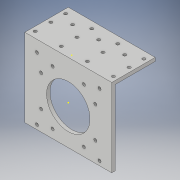
# Autodesk Inventor part: ousterholderm600V2
Saved by Autodesk Inventor 2019 (Build 230136000, 136)
## iProperties
Created: 2019-07-12
Part Number: ousterholderm600V2
Material: Generic
Document SubType Name: Modeling
Designer: Dell
Density: 1 g/cm^3
Appearance: Default
Author: Dell
Autodesk Inventor part; units mm, degrees
ref_plane "YZ Plane" through (0, 0, 0) normal (1, 0, 0) x (0, 1, 0)
ref_plane "XZ Plane" through (0, 0, 0) normal (0, 1, 0) x (-1, 0, 0)
ref_plane "XY Plane" through (0, 0, 0) normal (0, 0, 1) x (1, 0, 0)
sketch "Sketch3" plane through (0, 0, 0) normal (0, 0, 1) x (1, 0, 0)
  line L0 (-50, 45) -> (50, 45)
  line L1 (50, 45) -> (50, -45)
  line L2 (50, -45) -> (-50, -45)
  line L3 (-50, -45) -> (-50, 45)
  line L4 (-50, 45) -> (50, -45) construction
  line L5 (50, 45) -> (-50, -45) construction
  point P0 (0, 0)
  dimension "d4" = 100
  dimension "d5" = 90
  constraints: 12 end point, 2 midpoint, 2 parallel, 1 horizontal, 1 perpendicular
  measures "d4" distance of L1.end L2.end
  measures "d5" distance of L0.end L1.end
extrude "Extrusion2" add sketch "Sketch3" along normal blind 4
sketch "Sketch4" plane through (0, 0, 4) normal (0, 0, 1) x (1, 0, 0)
  point P0 (0, 0)
sketch "Sketch5" plane through (0, 0, 4) normal (0, 0, 1) x (1, 0, 0)
  line L0 (50, 45) -> (-50, 45) projected
  line L1 (50, 45) -> (-50, 45)
  line L2 (-50, 45) -> (-50, 41)
  line L3 (-50, 41) -> (50, 41)
  line L4 (50, 41) -> (50, 45)
  point P0 (0, 0)
  dimension "d8" = 4
  dimension "d9" = 100
  constraints: 8 end point, 2 parallel, 1 horizontal, 1 perpendicular
  measures "d8" distance of L1.end L2.end
  measures "d9" distance of L2.end L3.end
extrude "Extrusion3" add sketch "Sketch5" against normal blind 50
sketch "Sketch6" plane through (0, 0, 4) normal (0, 0, 1) x (1, 0, 0)
  line L0 (18, -31.18) -> (-18, -31.18)
  line L1 (-18, -31.18) -> (-18, 31.18)
  line L2 (-18, 31.18) -> (18, 31.18)
  line L3 (18, 31.18) -> (18, -31.18)
  line L4 (18, -31.18) -> (-18, 31.18) construction
  line L5 (-18, -31.18) -> (18, 31.18) construction
  circle A0 centre (-18, 31.18) radius 1.75
  circle A1 centre (18, 31.18) radius 1.75
  circle A2 centre (-18, -31.18) radius 1.75
  circle A3 centre (18, -31.18) radius 1.75
  line L6 (50, 45) -> (-50, 45) projected
  line L7 (0, 45) -> (0, -4)
  line L8 (-18, -35.18) -> (18, -35.18)
  line L9 (18, -35.18) -> (18, 27.18)
  line L10 (18, 27.18) -> (-18, 27.18)
  line L11 (-18, 27.18) -> (-18, -35.18)
  line L12 (-18, -35.18) -> (18, 27.18) construction
  line L13 (18, -35.18) -> (-18, 27.18) construction
  circle A4 centre (18, 27.18) radius 1.75
  circle A5 centre (-18, 27.18) radius 1.75
  circle A6 centre (18, -35.18) radius 1.75
  circle A7 centre (-18, -35.18) radius 1.75
  point P0 (0, 0)
  dimension "d14" = 3.5
  dimension "d15" = 3.5
  dimension "d16" = 3.5
  dimension "d17" = 3.5
  dimension "d89" = 49
  dimension "d90" = 62.36
  dimension "d91" = 3.5
  dimension "d92" = 3.5
  dimension "d93" = 3.5
  dimension "d94" = 3.5
  constraints: 26 end point, 8 centre point, 8 coincident, 5 midpoint, 4 parallel, 3 perpendicular, 2 horizontal, 1 point on line
  measures "d14" diameter of A0
  measures "d15" diameter of A1
  measures "d16" diameter of A2
  measures "d17" diameter of A3
  measures "d89" distance of L7.start L7.end
  measures "d90" distance of L10.end L8.start
  measures "d91" diameter of A4
  measures "d92" diameter of A5
  measures "d93" diameter of A6
  measures "d94" diameter of A7
extrude "Extrusion4" cut sketch "Sketch6" against normal blind 50 contours A5 L1 | L1 L10 A5 | A7 L8 L11 | L11 L8 A7 | A4 L10 L3 | L3 A4 | A6 L8 L9 | L9 L8 A6 | L1 A5 L10 | L10 A4 L3
sketch "Sketch7" plane through (0, 0, 4) normal (0, 0, 1) x (1, 0, 0)
  line L0 (31.18, -18) -> (-31.18, -18)
  line L1 (-31.18, -18) -> (-31.18, 18)
  line L2 (-31.18, 18) -> (31.18, 18)
  line L3 (31.18, 18) -> (31.18, -18)
  line L4 (31.18, -18) -> (-31.18, 18) construction
  line L5 (-31.18, -18) -> (31.18, 18) construction
  circle A0 centre (-31.18, 18) radius 1.75
  circle A1 centre (31.18, 18) radius 1.75
  circle A2 centre (-31.18, -18) radius 1.75
  circle A3 centre (31.18, -18) radius 1.75
  line L6 (50, 45) -> (-50, 45) projected
  line L7 (0, 45) -> (0, -4)
  line L8 (-31.18, -22) -> (31.18, -22)
  line L9 (31.18, -22) -> (31.18, 14)
  line L10 (31.18, 14) -> (-31.18, 14)
  line L11 (-31.18, 14) -> (-31.18, -22)
  line L12 (-31.18, -22) -> (31.18, 14) construction
  line L13 (31.18, -22) -> (-31.18, 14) construction
  circle A4 centre (31.18, 14) radius 1.75
  circle A5 centre (-31.18, 14) radius 1.75
  circle A6 centre (31.18, -22) radius 1.75
  circle A7 centre (-31.18, -22) radius 1.75
  point P0 (0, 0)
  dimension "d20" = 62.36
  dimension "d21" = 36
  dimension "d22" = 3.5
  dimension "d23" = 3.5
  dimension "d24" = 3.5
  dimension "d25" = 3.5
  dimension "d95" = 49
  dimension "d96" = 36
  dimension "d97" = 3.5
  dimension "d98" = 3.5
  dimension "d99" = 3.5
  dimension "d100" = 3.5
  constraints: 26 end point, 8 centre point, 8 coincident, 5 midpoint, 4 parallel, 2 horizontal, 2 perpendicular, 1 point on line, 1 vertical
  measures "d20" distance of L1.end L2.end
  measures "d21" distance of L0.end L1.end
  measures "d22" diameter of A0
  measures "d23" diameter of A1
  measures "d24" diameter of A2
  measures "d25" diameter of A3
  measures "d95" distance of L7.start L7.end
  measures "d96" distance of L8.end L9.end
  measures "d97" diameter of A4
  measures "d98" diameter of A5
  measures "d99" diameter of A6
  measures "d100" diameter of A7
extrude "Extrusion5" cut sketch "Sketch7" against normal blind 50 contours A5 L1 | L1 L10 A5 | A7 L8 L11 | L11 L8 A7 | A4 L10 L3 | L3 A4 | A6 L8 L9 | L9 L8 A6 | L1 A5 L10 | L10 A4 L3
sketch "Sketch8" plane through (0, 0, 4) normal (0, 0, 1) x (1, 0, 0)
  line L0 (50, 45) -> (-50, 45) projected
  line L1 (0, 45) -> (0, -4)
  circle A0 centre (0, -4) radius 25
  point P0 (0, 0)
  dimension "d101" = 49
  dimension "d102" = 50
  constraints: 2 end point, 1 centre point, 1 coincident, 1 midpoint, 1 vertical
  measures "d101" distance of L1.start L1.end
  measures "d102" diameter of A0
extrude "Extrusion6" cut sketch "Sketch8" against normal blind 43.6625
sketch "Sketch9" plane through (-50, 45, 4) normal (0, 1, 0) x (1, 0, 0)
  line L0 (0, 50) -> (0, 0) projected
  line L1 (100, 0) -> (0, 0) projected
  line L2 (0, 0) -> (35, 0)
  line L3 (35, 0) -> (35, 7)
  line L4 (35, 7) -> (0, 7)
  line L5 (0, 7) -> (0, 0)
  circle A0 centre (35, 7) radius 1.75
  line L6 (0, 0) -> (35, 0)
  line L7 (35, 0) -> (35, 25)
  line L8 (35, 25) -> (0, 25)
  line L9 (0, 25) -> (0, 0)
  circle A1 centre (35, 25) radius 1.75
  point P0 (50, 4)
  dimension "d31" = 35
  dimension "d32" = 7
  dimension "d36" = 3.5
  dimension "d39" = 25
  dimension "d40" = 3.5
  constraints: 16 end point, 5 equal length, 2 centre point, 2 coincident, 2 perpendicular, 1 point on line
  measures "d31" distance of L3.end L4.end
  measures "d32" distance of L2.end L3.end
  measures "d36" diameter of A0
  measures "d39" distance of L7.end L2.end
  measures "d40" diameter of A1
sketch "Sketch10" plane through (-50, 45, 4) normal (0, 1, 0) x (1, 0, 0)
  line L0 (100, 4) -> (100, 0) projected
  line L1 (100, 0) -> (0, 0) projected
  line L2 (100, 0) -> (65, 0)
  line L3 (65, 0) -> (65, 7)
  line L4 (65, 7) -> (100, 7)
  line L5 (100, 7) -> (100, 0)
  circle A0 centre (65, 7) radius 1.75
  line L6 (100, 0) -> (65, 0)
  line L7 (65, 0) -> (65, 25)
  line L8 (65, 25) -> (100, 25)
  line L9 (100, 25) -> (100, 0)
  line L10 (75, 0) -> (25, 0) projected
  circle A1 centre (65, 25) radius 1.75
  point P0 (50, 4)
  dimension "d33" = 35
  dimension "d34" = 7
  dimension "d35" = 3.5
  dimension "d37" = 25
  dimension "d38" = 3.5
  constraints: 16 end point, 4 parallel, 2 centre point, 2 coincident, 2 perpendicular, 1 collinear, 1 point on line
  measures "d33" distance of L0.end L2.end
  measures "d34" distance of L2.end L3.end
  measures "d35" diameter of A0
  measures "d37" distance of L2.end L7.end
  measures "d38" diameter of A1
sketch "Sketch11" plane through (-50, 45, 4) normal (0, 1, 0) x (1, 0, 0)
  point P0 (50, 4)
extrude "Extrusion7" cut sketch "Sketch9" against normal blind 43.6625 contours A1 L7 L8 | L8 L7 A1 | A0 L7 L4 | L4 L3 A0 | L7 A0 L3
extrude "Extrusion8" cut sketch "Sketch10" against normal blind 43.6625 contours A0 L3 L4 | L4 L7 A0 | L3 A0 L7 | A1 L7 L8 | L8 L7 A1
sketch "Sketch12" plane through (-50, 45, 4) normal (0, 1, 0) x (1, 0, 0)
  line L0 (0, 0) -> (100, 0) projected
  line L1 (0, 0) -> (5, 0)
  line L2 (5, 0) -> (5, 7)
  line L3 (5, 7) -> (0, 7)
  line L4 (0, 7) -> (0, 0)
  line L5 (100, 0) -> (0, 0) projected
  line L6 (0, 0) -> (5, 0)
  line L7 (5, 0) -> (5, 25)
  line L8 (5, 25) -> (0, 25)
  line L9 (0, 25) -> (0, 0)
  circle A0 centre (5, 7) radius 1.75
  circle A1 centre (5, 25) radius 1.75
  point P0 (50, 4)
  dimension "d45" = 5
  dimension "d46" = 7
  dimension "d47" = 25
  dimension "d48" = 3.5
  dimension "d49" = 3.5
  constraints: 16 end point, 4 parallel, 2 centre point, 2 coincident, 2 perpendicular, 1 collinear, 1 point on line
  measures "d45" distance of L0.start L1.end
  measures "d46" distance of L2.end L1.end
  measures "d47" distance of L7.end L1.end
  measures "d48" diameter of A0
  measures "d49" diameter of A1
extrude "Extrusion9" cut sketch "Sketch12" against normal blind 43.6625 contours A0 L3 L2 | L2 L7 A0 | A0 L7 L3 | A1 L7 L8 | L8 L7 A1
sketch "Sketch13" plane through (-50, 45, 4) normal (0, 1, 0) x (1, 0, 0)
  line L0 (0, 0) -> (100, 0) projected
  line L1 (100, 0) -> (95, 0)
  line L2 (95, 0) -> (95, 7)
  line L3 (95, 7) -> (100, 7)
  line L4 (100, 7) -> (100, 0)
  line L5 (100, 0) -> (95, 0)
  line L6 (95, 0) -> (95, 25)
  line L7 (95, 25) -> (100, 25)
  line L8 (100, 25) -> (100, 0)
  circle A0 centre (95, 25) radius 1.75
  circle A1 centre (95, 7) radius 1.75
  point P0 (50, 4)
  dimension "d52" = 5
  dimension "d53" = 7
  dimension "d54" = 25
  dimension "d55" = 3.5
  dimension "d56" = 3.5
  constraints: 16 end point, 4 parallel, 2 centre point, 2 coincident, 2 perpendicular, 1 collinear, 1 point on line
  measures "d52" distance of L0.end L1.end
  measures "d53" distance of L1.end L2.end
  measures "d54" distance of L1.end L6.end
  measures "d55" diameter of A0
  measures "d56" diameter of A1
extrude "Extrusion10" cut sketch "Sketch13" against normal blind 43.6625 contours A1 L6 L2 | L2 L3 A1 | L6 A1 L3 | A0 L7 L6 | L6 L7 A0
sketch "Sketch14" plane through (-50, 45, 4) normal (0, 1, 0) x (1, 0, 0)
  point P0 (50, 4)
sketch "Sketch15" plane through (-50, 45, 4) normal (0, 1, 0) x (1, 0, 0)
  line L0 (0, 50) -> (100, 50) projected
  line L1 (0, 50) -> (50, 50)
  line L2 (50, 50) -> (50, 42)
  line L3 (50, 42) -> (0, 42)
  line L4 (0, 42) -> (0, 50)
  line L5 (0, 50) -> (35, 50)
  line L6 (35, 50) -> (35, 42)
  line L7 (35, 42) -> (0, 42)
  line L8 (0, 42) -> (0, 50)
  line L9 (0, 4) -> (0, 50) projected
  line L10 (0, 50) -> (5, 50)
  line L11 (5, 50) -> (5, 42)
  line L12 (5, 42) -> (0, 42)
  line L13 (0, 42) -> (0, 50)
  line L14 (100, 4) -> (100, 50) projected
  line L15 (100, 50) -> (95, 50)
  line L16 (95, 50) -> (95, 42)
  line L17 (95, 42) -> (100, 42)
  line L18 (100, 42) -> (100, 50)
  line L19 (100, 50) -> (0, 50) projected
  line L20 (100, 50) -> (65, 50)
  line L21 (65, 50) -> (65, 42)
  line L22 (65, 42) -> (100, 42)
  line L23 (100, 42) -> (100, 50)
  circle A0 centre (5, 42) radius 1.75
  circle A1 centre (35, 42) radius 1.75
  circle A2 centre (65, 42) radius 1.75
  circle A3 centre (95, 42) radius 1.75
  point P0 (50, 4)
  dimension "d60" = 8
  dimension "d61" = 35
  dimension "d62" = 5
  dimension "d63" = 5
  dimension "d64" = 35
  dimension "d66" = 3.5
  dimension "d67" = 3.5
  dimension "d68" = 3.5
  dimension "d69" = 3.5
  constraints: 40 end point, 10 parallel, 5 perpendicular, 4 centre point, 4 coincident, 4 point on line, 1 midpoint
  measures "d60" distance of L1.end L2.end
  measures "d61" distance of L0.start L5.end
  measures "d62" distance of L0.start L10.end
  measures "d63" distance of L0.end L15.end
  measures "d64" distance of L0.end L20.end
  measures "d66" diameter of A0
  measures "d67" diameter of A1
  measures "d68" diameter of A2
  measures "d69" diameter of A3
extrude "Extrusion11" cut sketch "Sketch15" against normal blind 43.6625 contours A0 L3 L11 | L11 L3 A0 | L3 A0 | A1 L3 L6 | L6 L3 A1 | L3 A1 | A2 L22 L21 | L21 L22 A2 | A3 L17 L16 | L16 L22 A3 | L17 A3 L22
sketch "Sketch16" plane through (-50, 45, 4) normal (0, 1, 0) x (1, 0, 0)
  line L0 (100, 50) -> (0, 50) projected
  line L1 (0, 50) -> (20, 50)
  line L2 (20, 50) -> (20, 35)
  line L3 (20, 35) -> (0, 35)
  line L4 (0, 35) -> (0, 50)
  line L5 (0, 50) -> (0, 0) projected
  line L6 (0, 50) -> (50, 50)
  line L7 (50, 50) -> (50, 35)
  line L8 (50, 35) -> (0, 35)
  line L9 (0, 35) -> (0, 50)
  line L10 (100, 4) -> (100, 50) projected
  line L11 (100, 50) -> (80, 50)
  line L12 (80, 50) -> (80, 35)
  line L13 (80, 35) -> (100, 35)
  line L14 (100, 35) -> (100, 50)
  circle A0 centre (20, 35) radius 1.75
  circle A1 centre (50, 35) radius 1.75
  circle A2 centre (80, 35) radius 1.75
  point P0 (50, 4)
  dimension "d72" = 20
  dimension "d73" = 15
  dimension "d74" = 50
  dimension "d75" = 20
  dimension "d76" = 3.5
  dimension "d77" = 3.5
  dimension "d78" = 3.5
  constraints: 24 end point, 6 parallel, 3 centre point, 3 coincident, 3 horizontal, 3 perpendicular, 1 point on line
  measures "d72" distance of L2.end L3.end
  measures "d73" distance of L1.end L2.end
  measures "d74" distance of L7.end L8.end
  measures "d75" distance of L13.end L12.end
  measures "d76" diameter of A0
  measures "d77" diameter of A1
  measures "d78" diameter of A2
extrude "Extrusion12" cut sketch "Sketch16" against normal blind 10 contours A2 L13 L12 | L12 L13 A2 | A1 L8 L7 | L7 L8 A1 | A0 L8 L2 | L2 L3 A0 | L8 A0 L3
sketch "Sketch17" plane through (0, 0, 4) normal (0, 0, 1) x (1, 0, 0)
  line L0 (36, -36) -> (-36, -36)
  line L1 (-36, -36) -> (-36, 36)
  line L2 (-36, 36) -> (36, 36)
  line L3 (36, 36) -> (36, -36)
  line L4 (36, -36) -> (-36, 36) construction
  line L5 (-36, -36) -> (36, 36) construction
  circle A0 centre (-36, 36) radius 1.75
  circle A1 centre (36, 36) radius 1.75
  circle A2 centre (36, -36) radius 1.75
  circle A3 centre (-36, -36) radius 1.75
  line L6 (50, 45) -> (-50, 45) projected
  line L7 (0, 45) -> (0, -4)
  line L8 (-36, -40) -> (36, -40)
  line L9 (36, -40) -> (36, 32)
  line L10 (36, 32) -> (-36, 32)
  line L11 (-36, 32) -> (-36, -40)
  line L12 (-36, -40) -> (36, 32) construction
  line L13 (36, -40) -> (-36, 32) construction
  circle A4 centre (36, 32) radius 1.75
  circle A5 centre (36, -40) radius 1.75
  circle A6 centre (-36, -40) radius 1.75
  circle A7 centre (-36, 32) radius 1.75
  point P0 (0, 0)
  dimension "d81" = 72
  dimension "d82" = 72
  dimension "d83" = 3.5
  dimension "d84" = 3.5
  dimension "d85" = 3.5
  dimension "d86" = 3.5
  dimension "d103" = 49
  dimension "d104" = 72
  dimension "d105" = 3.5
  dimension "d106" = 3.5
  dimension "d107" = 3.5
  dimension "d108" = 3.5
  constraints: 26 end point, 8 centre point, 8 coincident, 5 midpoint, 4 parallel, 3 perpendicular, 2 horizontal, 1 point on line
  measures "d81" distance of L1.end L2.end
  measures "d82" distance of L0.end L1.end
  measures "d83" diameter of A0
  measures "d84" diameter of A1
  measures "d85" diameter of A2
  measures "d86" diameter of A3
  measures "d103" distance of L7.start L7.end
  measures "d104" distance of L10.end L8.start
  measures "d105" diameter of A4
  measures "d106" diameter of A5
  measures "d107" diameter of A6
  measures "d108" diameter of A7
extrude "Extrusion13" cut sketch "Sketch17" against normal blind 10 contours A7 L1 | L1 L10 A7 | A6 L8 L11 | L11 L8 A6 | A4 L10 L3 | L3 A4 | A5 L8 L9 | L9 L8 A5 | L1 A7 L10 | L10 A4 L3
body "Solid2"
